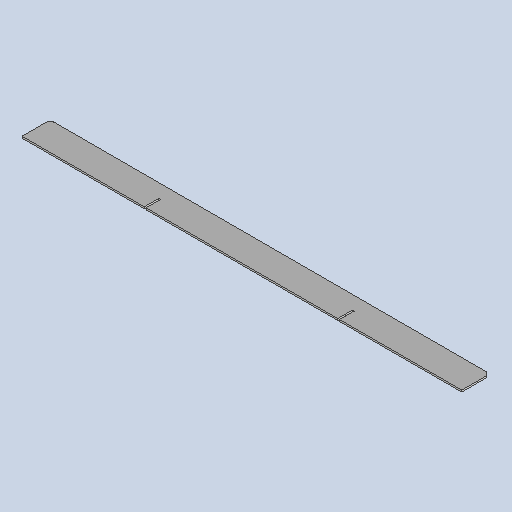
# Autodesk Inventor part: MSC 109 RIB CONE
Saved by Autodesk Inventor 2025 (Build 290162010, 162A)
## iProperties
Created: 2024-06-26
Part Number: MSC 109 RIB CONE
Material: Stainless Steel
Document SubType Name: Sheet Metal
Designer: pokla
Density: 8 g/cm^3
Sheet Metal Rule: AISI304 3mm Die 32
Appearance: Default
Stock Number: МОО 109 шпангоут конус
Mass: 931.267 g
Surface Area: 828.765 cm^2
Volume: 116.408 cm^3
Flat Pattern Width: 5 cm
Flat Pattern Length: 78 cm
Flat Pattern Area: 390 cm^2
Sheet Metal Width: 50,000 mm
Sheet Metal Length: 780,000 mm
Sheet Metal Area: 39000,000 mm^2
Author: pokla
Autodesk Inventor part; units mm, degrees
ref_plane "YZ Plane" through (0, 0, 0) normal (1, 0, 0) x (0, 1, 0)
ref_plane "XZ Plane" through (0, 0, 0) normal (0, 1, 0) x (-1, 0, 0)
ref_plane "XY Plane" through (0, 0, 0) normal (0, 0, 1) x (1, 0, 0)
sketch "Sketch1" plane through (0, 0, 0) normal (0, 0, 1) x (1, 0, 0)
  line L0 (-390, 50) -> (390, 50)
  line L1 (390, 50) -> (390, 0)
  line L2 (390, 0) -> (-390, 0)
  line L3 (-390, 0) -> (-390, 50)
  circle A0 centre (-390, 0) radius 25
  circle A1 centre (390, 0) radius 25
  point P0 (0, 0)
  point P1 (0, 0)
  point P2 (-390, 25)
  point P3 (-365, 0)
  point P4 (365, 0)
  point P5 (390, 25)
  dimension "d16" = 50
  dimension "d17" = 780
  dimension "d18" = 50
  dimension "d19" = 50
  measures "d16" distance of L0.end L1.end
  measures "d17" distance of L0.start L0.end
  measures "d18" diameter of A0
  measures "d19" diameter of A1
extrude "Plate2" add sketch "Sketch1" against normal blind 3 contours L0 L1 A1 L2 A0 L3 | A0 L2 L3 | L1 L2 A1 picked at (-378.289, 11.711) picked at (388.1457, 16.4577)
sketch "Sketch2" plane through (0, 0, 0) normal (0, 0, 1) x (1, 0, 0)
  line L0 (390, 50) -> (-390, 50) projected
  line L1 (171.55, 50) -> (171.55, 0) construction
  line L2 (-390, 0) -> (390, 0) projected
  line L3 (170, 26) -> (173.1, 26)
  line L4 (173.1, 26) -> (173.1, 0)
  line L5 (173.1, 0) -> (170, 0)
  line L6 (170, 0) -> (170, 26)
  line L7 (-171.55, 0) -> (-171.55, 50) construction
  line L8 (-173.1, 26) -> (-170, 26)
  line L9 (-170, 26) -> (-170, 0)
  line L10 (-170, 0) -> (-173.1, 0)
  line L11 (-173.1, 0) -> (-173.1, 26)
  line L12 (0, 0) -> (0, 50)
  point P0 (0, 0)
  point P1 (170, 0)
  point P2 (173.1, 0)
  point P3 (-173.1, 0)
  point P4 (-170, 0)
  dimension "d27" = 26
  dimension "d28" = 3.1
  dimension "d34" = 340
  constraints: 22 end point, 5 midpoint, 4 parallel, 4 point on line, 3 perpendicular, 2 equal length, 2 horizontal, 1 vertical, 1 other
  measures "d27" distance of L10.end L8.start
  measures "d28" distance of L9.end L10.end
  measures "d34" distance between parallel lines of L6 L9
extrude "Extrusion1" cut sketch "Sketch2" against normal blind 10
sketch "Sketch4" plane through (0, 0, -3) normal (0, 0, -1) x (-1, 0, 0)
  line L0 (-62.455, 14.7345) -> (-62.455, 33.3208) construction
  line L1 (-62.455, 33.3208) -> (59.5733, 33.3208) construction
  line L2 (59.5733, 33.3208) -> (59.5733, 14.7345) construction
  line L3 (59.5733, 14.7345) -> (-62.455, 14.7345) construction
  point P0 (0, 0)
  constraints: 2 other
mark "Mark1"
chamfer "Corner Chamfer1" distance 6 angle 45 2 edges at (390, 50, -1.5) (-390, 50, -1.5)
equation "\"d27\" = d23"
equation "\"d20\" = Thickness"
equation "\"BendReliefWidth\" = Thickness"
equation "\"BendReliefDepth\" = 0.5 * Thickness"
equation "\"CornerReliefSize\" = 4 * Thickness"
equation "\"MinimumRemnant\" = 2 * Thickness"
equation "\"TransitionRadius\" = BendRadius"
equation "\"JacobiRadiusSize\" = BendRadius"
equation "\"GapSize\" = Thickness"
equation "\"d23\" = 26"
equation "\"Thickness\" = 3"
equation "\"BendRadius\" = 5"
body "Solid2"
